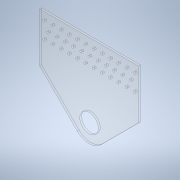
# Autodesk Inventor part: Krystal Plate
Saved by Autodesk Inventor 2020 (Build 240168000, 168)
## iProperties
Created: 2020-02-06
Part Number: Krystal Plate
Material: Polycarbonate, Clear
Document SubType Name: Modeling
Designer: aidan
Density: 1.2 g/cm^3
Appearance: Polycarbonate - Clear
Author: aidan
Autodesk Inventor part; units mm, degrees
ref_plane "YZ Plane" through (0, 0, 0) normal (1, 0, 0) x (0, 1, 0)
ref_plane "XZ Plane" through (0, 0, 0) normal (0, 1, 0) x (-1, 0, 0)
ref_plane "XY Plane" through (0, 0, 0) normal (0, 0, 1) x (1, 0, 0)
sketch "Sketch1" plane through (0, 0, 0) normal (0, 0, 1) x (1, 0, 0)
  line L0 (-63.1045, 37.3635) -> (89.2955, 37.3635)
  line L1 (89.2955, 37.3635) -> (89.2955, -38.8365)
  line L2 (-63.1045, -38.8365) -> (-63.1045, 37.3635)
  line L3 (-63.1045, -38.8365) -> (13.0955, -115.0365)
  line L4 (13.0955, -115.0365) -> (89.2955, -38.8365)
  line L5 (13.0955, -115.0365) -> (13.0955, 37.3635) construction
  point P0 (0, 0)
  dimension "d0" = 152.4
  dimension "d1" = 76.2
  dimension "d2" = 76.2
  constraints: 12 end point, 2 perpendicular, 1 horizontal, 1 midpoint, 1 parallel, 1 vertical
  measures "d0" distance of L0.start L0.end
  measures "d1" distance of L0.end L1.end
  measures "d2" horizontal distance of L1.end L3.end
extrude "Extrusion1" add sketch "Sketch1" along normal blind 2.9972
sketch "Sketch2" plane through (0, 0, 2.9972) normal (0, 0, 1) x (1, 0, 0)
  line L0 (-63.1045, 37.3635) -> (-63.1045, -38.8365) projected
  line L1 (-63.1045, 24.6635) -> (89.2955, 24.6635) construction
  line L2 (89.2955, -38.8365) -> (89.2955, 37.3635) projected
  line L3 (89.2955, 11.9635) -> (-63.1045, 11.9635) construction
  line L4 (-63.1045, -0.7365) -> (89.2955, -0.7365) construction
  line L5 (89.2955, 37.3635) -> (-63.1045, 37.3635) projected
  circle A0 centre (-56.7545, 24.6635) radius 1.7272
  circle A1 centre (-50.4045, 11.9635) radius 1.7272
  circle A2 centre (-56.7545, -0.7365) radius 1.7272
  point P0 (0, 0)
  dimension "d5" = 12.7
  dimension "d6" = 12.7
  dimension "d7" = 12.7
  dimension "d8" = 3.4544
  dimension "d9" = 6.35
  dimension "d10" = 6.35
  dimension "d11" = 12.7
  constraints: 6 end point, 6 point on line, 3 centre point, 2 equal radius, 2 horizontal
  measures "d5" distance between parallel lines of L5 L1
  measures "d6" distance between parallel lines of L3 L1
  measures "d7" distance between parallel lines of L3 L4
  measures "d8" diameter of A0
  measures "d9" distance from line of L0 A0.centre
  measures "d10" distance from line of L0 A2.centre
  measures "d11" distance from line of L0 A1.centre
extrude "Extrusion2" cut sketch "Sketch2" against normal through all contours A0 | A2
extrude "Extrusion3" cut sketch "Sketch2" against normal through all contours A1
pattern_linear "Rectangular Pattern1" count 12 spacing 12.7 along (1, 0, 0) of "Extrusion2"
pattern_linear "Rectangular Pattern2" count 11 spacing 12.7 along (1, 0, 0) of "Extrusion3"
sketch "Sketch3" plane through (0, 0, 2.9972) normal (0, 0, 1) x (1, 0, 0)
  circle A0 centre (13.0955, -76.9365) radius 14.2875
  line L0 (-63.1045, -38.8365) -> (13.0955, -115.0365) projected
  line L1 (13.0955, -76.9365) -> (13.0955, -115.0365) construction
  point P0 (0, 0)
  dimension "d22" = 28.575
  dimension "d23" = 38.1
  constraints: 2 end point, 1 centre point, 1 vertical
  measures "d22" diameter of A0
  measures "d23" distance of L1.start L0.end
extrude "Extrusion4" cut sketch "Sketch3" against normal through all
fillet "Fillet1" radius 25.4 1 edges at (13.0955, -115.0365, 1.4986)
body "Solid1"
